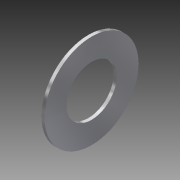
# Autodesk Inventor part: 5909K44
Saved by Autodesk Inventor 2013 (Build 170138000, 138)
## iProperties
Created: 2013-04-01
Part Number: 5909K44
Material: Generic
Document SubType Name: Modeling
Designer: mvarma
Density: 1 g/cm^3
Translation Standard: STEP AP203
FileName: 5909K44.step
PreProcessor: SolidWorks 2007
PostProcessor: Build: 138, Release: 2013 RTM - Date: Thu 03/01/2012
Sent Units: inch
Uncertainty: 1e-05
Author: mvarma
Autodesk Inventor part; units mm, degrees
ref_plane "YZ Plane" through (0, 0, 0) normal (1, 0, 0) x (0, 1, 0)
ref_plane "XZ Plane" through (0, 0, 0) normal (0, 1, 0) x (-1, 0, 0)
ref_plane "XY Plane" through (0, 0, 0) normal (0, 0, 1) x (1, 0, 0)
sketch "Sketch2" plane through (0, 0, 0) normal (1, 0, 0) x (0, 1, 0)
  circle A0 centre (0, 0) radius 6.35
  circle A1 centre (0, 0) radius 11.9062
  dimension "d0" = 12.7
  dimension "d2" = 23.8125
  constraints: 2 centre point, 2 coincident
  measures "d0" diameter of A0
  measures "d2" diameter of A1
extrude "Extrusion1" add sketch "Sketch2" along normal blind 0.7937
body "Solid2"
